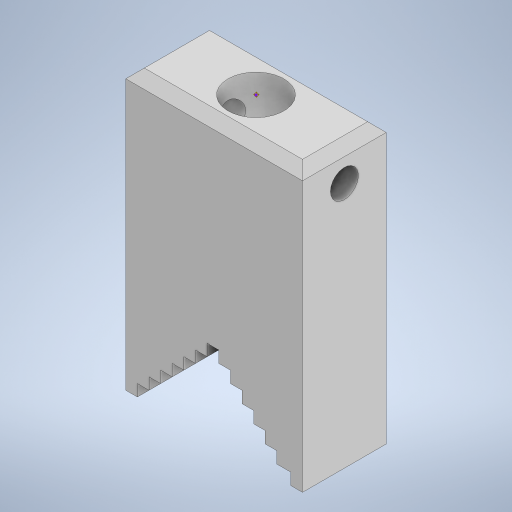
# Autodesk Inventor part: Machoire
Saved by Autodesk Inventor 2023.2 (Build 272271030, 271C)
## iProperties
Created: 2023-03-02
Part Number: Machoire
Material: Generic
Document SubType Name: Modeling
Designer: Luis Valente
Density: 1 g/cm^3
Appearance: Default
Author: Luis Valente
Autodesk Inventor part; units mm, degrees
ref_plane "YZ Plane" through (0, 0, 0) normal (1, 0, 0) x (0, 1, 0)
ref_plane "XZ Plane" through (0, 0, 0) normal (0, 1, 0) x (-1, 0, 0)
ref_plane "XY Plane" through (0, 0, 0) normal (0, 0, 1) x (1, 0, 0)
sketch "Sketch1" plane through (0, 0, 0) normal (0, 0, 1) x (1, 0, 0)
  line L0 (0, 0) -> (38, 0)
  line L1 (38, 0) -> (38, 60)
  line L2 (38, 60) -> (0, 60)
  line L3 (0, 60) -> (0, 0)
  dimension "d0" = 38
  dimension "d1" = 60
  constraints: 8 end point, 2 parallel, 1 horizontal, 1 perpendicular
  measures "d0" distance of L2.end L1.end
  measures "d1" distance of L1.end L0.end
extrude "Extrusion1" add sketch "Sketch1" along normal blind 18
sketch "Sketch2" plane through (0, 0, 18) normal (0, 0, 1) x (1, 0, 0)
  line L0 (0, 60) -> (0, 0) projected
  line L1 (0, 0) -> (2.5, 0)
  line L2 (0, 0) -> (38, 0) projected
  line L3 (2.5, 0) -> (2.5, 2.5)
  line L4 (2.5, 2.5) -> (5, 2.5)
  line L5 (5, 2.5) -> (5, 5)
  line L6 (5, 5) -> (7.5, 5)
  line L7 (7.5, 5) -> (7.5, 7.5)
  line L8 (7.5, 7.5) -> (10, 7.5)
  line L9 (10, 7.5) -> (10, 10)
  line L10 (10, 10) -> (12.5, 10)
  line L11 (12.5, 10) -> (12.5, 12.5)
  line L12 (12.5, 12.5) -> (15, 12.5)
  line L13 (15, 12.5) -> (15, 15)
  line L14 (15, 15) -> (17.5, 15)
  line L15 (17.5, 15) -> (17.5, 17.5)
  line L16 (17.5, 17.5) -> (18.75, 17.5)
  line L17 (38, 0) -> (35.5, 0)
  line L18 (35.5, 0) -> (35.5, 2.5)
  line L19 (35.5, 2.5) -> (32.5, 2.5)
  line L20 (32.5, 2.5) -> (32.5, 5)
  line L21 (32.5, 5) -> (30, 5)
  line L22 (30, 5) -> (30, 7.5)
  line L23 (30, 7.5) -> (27.5, 7.5)
  line L24 (27.5, 7.5) -> (27.5, 10)
  line L25 (27.5, 10) -> (25, 10)
  line L26 (25, 10) -> (25, 12.5)
  line L27 (25, 12.5) -> (22.5, 12.5)
  line L28 (22.5, 12.5) -> (22.5, 15)
  line L29 (22.5, 15) -> (20, 15)
  line L30 (20, 15) -> (20, 17.5)
  line L31 (20, 17.5) -> (18.75, 17.5)
  dimension "d27" = 2.5
  dimension "d28" = 2.5
  constraints: 60 end point, 11 perpendicular, 2 horizontal, 1 point on line, 1 vertical
  measures "d27" distance of L0.end L1.end
  measures "d28" distance of L30.end L15.end
extrude "Extrusion2" cut sketch "Sketch2" against normal blind 18
sketch "Sketch3" plane through (0, 0, 0) normal (-1, 0, 0) x (0, 0, 1)
  line L0 (0, 60) -> (18, 60) projected
  line L1 (0, 60) -> (0, 53)
  line L2 (0, 60) -> (0, 0) projected
  line L3 (0, 53) -> (9, 53)
  line L4 (18, 60) -> (18, 0) projected
  circle A0 centre (9, 53) radius 3
  dimension "d31" = 7
  dimension "d32" = 9
  dimension "d33" = 6
  constraints: 4 end point, 1 centre point, 1 coincident, 1 perpendicular, 1 point on line
  measures "d31" distance of L0.start L1.end
  measures "d32" distance of L1.end L3.end
  measures "d33" diameter of A0
extrude "Extrusion3" cut sketch "Sketch3" against normal blind 38
sketch "Sketch4" plane through (0, 60, 0) normal (0, 1, 0) x (1, 0, 0)
  point P0 (19, -9)
hole "Hole1" at (19, 60, 9) direction (0, -1, 0) diameter 12 depth 10 tip angle 120
chamfer "Chamfer1" distance 2 angle 45 4 edges at (19, 60, 18) (38, 60, 9) (19, 60, 0) (0, 60, 9) measured on face at (4.3479, 60, 9.2411)
body "Solid1"
